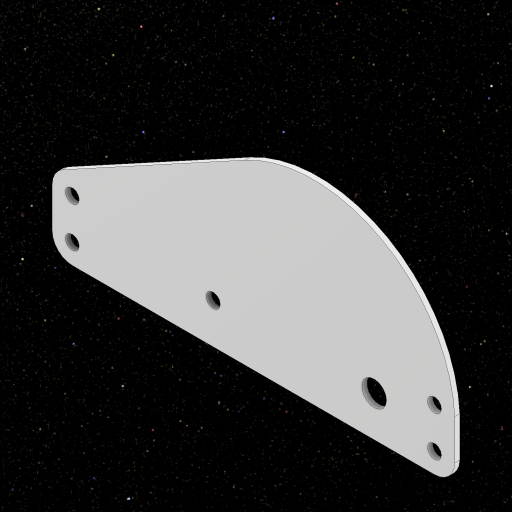
# Autodesk Inventor part: intake_sled
Saved by Autodesk Inventor 2024 (Build 280153000, 153)
## iProperties
Created: 2024-02-24
Part Number: intake_sled
Material: Acetal Resin, White
Document SubType Name: Modeling
Designer: Averey Ku
Density: 1.425 g/cm^3
Appearance: Smooth - White
Author: Averey Ku
Autodesk Inventor part; units mm, degrees
ref_plane "YZ Plane" through (0, 0, 0) normal (1, 0, 0) x (0, 1, 0)
ref_plane "XZ Plane" through (0, 0, 0) normal (0, 1, 0) x (-1, 0, 0)
ref_plane "XY Plane" through (0, 0, 0) normal (0, 0, 1) x (1, 0, 0)
sketch "main" plane through (0, 0, 0) normal (0, 0, 1) x (1, 0, 0)
  circle A0 centre (50.5981, -28.4488) radius 2.1844
  line L0 (-66.7437, -10.1747) -> (-9.1578, 21.251)
  line L1 (50.5981, -34.7988) -> (-63.7019, -34.7988)
  circle A1 centre (50.5981, -15.7488) radius 2.1844
  arc A2 (50.5981, -34.7988) -> (56.9481, -28.4488) centre (50.5981, -28.4488) ccw
  line L2 (56.9481, -28.4488) -> (56.9481, -15.7488)
  arc A3 (56.9481, -15.7488) -> (56.9038, -14.9999) centre (50.5981, -15.7488) ccw
  arc A4 (56.9481, -15.7488) -> (-9.1578, 21.251) centre (12.2713, -18.0166) ccw
  circle A5 centre (31.5481, -22.0988) radius 3.9
  circle A6 centre (-19.2519, -22.0988) radius 2.2479
  circle A7 centre (-63.7019, -28.4488) radius 2.1844
  circle A8 centre (-63.7019, -15.7488) radius 2.1844
  arc A9 (-66.7437, -10.1747) -> (-70.0519, -15.7488) centre (-63.7019, -15.7488) ccw
  line L3 (-70.0519, -28.4488) -> (-70.0519, -15.7488)
  arc A10 (-70.0519, -28.4488) -> (-63.7019, -34.7988) centre (-63.7019, -28.4488) ccw
  point P0 (-3.3794, -19.3684)
  dimension "d0" = 7.8
  dimension "d1" = 4.4958
  measures "d0" diameter of A5
  measures "d1" diameter of A6
sketch "Sketch1" plane through (0, 0, 0) normal (0, 0, 1) x (1, 0, 0)
  circle A0 centre (0, 0) radius 2.1844
  line L0 (-117.3419, 18.274) -> (-59.7559, 49.6998)
  line L1 (0, -6.35) -> (-114.3, -6.35)
  circle A1 centre (0, 12.7) radius 2.1844
  arc A2 (0, -6.35) -> (6.35, 0) centre (0, 0) ccw
  line L2 (6.35, 0) -> (6.35, 12.7)
  arc A3 (6.35, 12.7) -> (6.3057, 13.4489) centre (0, 12.7) ccw
  arc A4 (6.35, 12.7) -> (-59.7559, 49.6998) centre (-38.3268, 10.4321) ccw
  circle A5 centre (-19.05, 6.35) radius 3.9
  circle A6 centre (-69.85, 6.35) radius 2.2479
  circle A7 centre (-114.3, 0) radius 2.1844
  circle A8 centre (-114.3, 12.7) radius 2.1844
  arc A9 (-117.3419, 18.274) -> (-120.65, 12.7) centre (-114.3, 12.7) ccw
  line L3 (-120.65, 0) -> (-120.65, 12.7)
  arc A10 (-120.65, 0) -> (-114.3, -6.35) centre (-114.3, 0) ccw
  constraints: 1 other
extrude "Extrusion1" add sketch "Sketch1" along normal blind 1.5875 contours L0 A4 L2 A2 L1 A10 L3 A9
body "Solid1"
